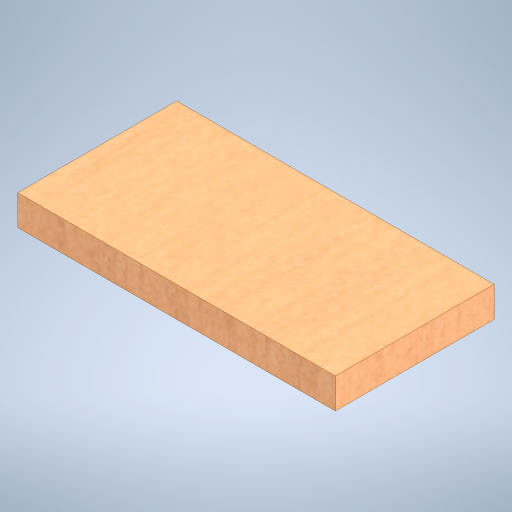
# Autodesk Inventor part: Querseite_Konsole
Saved by Autodesk Inventor 2024 (Build 280153000, 153)
## iProperties
Created: 2024-05-02
Part Number: Querseite_Konsole
Material: Holz (Kirsche)
Document SubType Name: Modeling
Designer: haniv
Density: 0.63 g/cm^3
Appearance: Kirsche - natur - schwacher Glanz
Author: haniv
Autodesk Inventor part; units mm, degrees
ref_plane "YZ Plane" through (0, 0, 0) normal (1, 0, 0) x (0, 1, 0)
ref_plane "XZ Plane" through (0, 0, 0) normal (0, 1, 0) x (-1, 0, 0)
ref_plane "XY Plane" through (0, 0, 0) normal (0, 0, 1) x (1, 0, 0)
sketch "Skizze1" plane through (0, 0, 0) normal (0, 0, 1) x (1, 0, 0)
  line L0 (-63, 31.5) -> (63, 31.5)
  line L1 (63, 31.5) -> (63, -31.5)
  line L2 (63, -31.5) -> (-63, -31.5)
  line L3 (-63, -31.5) -> (-63, 31.5)
  point P0 (0, 0)
  point P1 (0, 31.5)
  point P2 (-63, 0)
  dimension "d0" = 126
  dimension "d1" = 63
  constraints: 8 end point, 2 midpoint, 2 parallel, 1 horizontal, 1 horizontal alignment, 1 perpendicular, 1 vertical alignment
  measures "d0" distance of L1.end L2.end
  measures "d1" distance of L0.end L1.end
extrude "Extrusion1" add sketch "Skizze1" along normal blind 12
